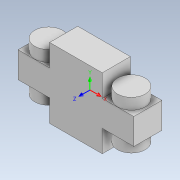
# Autodesk Inventor part: body_inventor
Saved by Autodesk Inventor 2020 (Build 240168000, 168)
## iProperties
Created: 2021-01-07
Part Number: body_inventor
Material: Generic
Document SubType Name: Modeling
Designer: DELL
Density: 1 g/cm^3
Appearance: Default
Author: DELL
Autodesk Inventor part; units mm, degrees
ref_plane "YZ Plane" through (0, 0, 0) normal (1, 0, 0) x (0, 1, 0)
ref_plane "XZ Plane" through (0, 0, 0) normal (0, 1, 0) x (-1, 0, 0)
ref_plane "XY Plane" through (0, 0, 0) normal (0, 0, 1) x (1, 0, 0)
sketch "Sketch4" plane through (0, 0, 0) normal (0, 0, 1) x (1, 0, 0)
  line L0 (75, -100) -> (-75, -100)
  line L1 (-75, -100) -> (-75, 100)
  line L2 (-75, 100) -> (75, 100)
  line L3 (75, 100) -> (75, -100)
  line L4 (75, -100) -> (-75, 100) construction
  line L5 (-75, -100) -> (75, 100) construction
  line L6 (165, -37) -> (-165, -37)
  line L7 (-165, -37) -> (-165, 37)
  line L8 (-165, 37) -> (165, 37)
  line L9 (165, 37) -> (165, -37)
  line L10 (165, -37) -> (-165, 37) construction
  line L11 (-165, -37) -> (165, 37) construction
  point P0 (0, 0)
  point P1 (0, 0)
  point P2 (0, 0)
  point P3 (75, 37)
  point P4 (-75, 37)
  point P5 (-75, -37)
  point P6 (75, -37)
  dimension "d17" = 74
  dimension "d18" = 330
  dimension "d19" = 150
  dimension "d20" = 200
  constraints: 24 end point, 5 midpoint, 4 parallel, 2 horizontal, 2 perpendicular, 1 coincident
  measures "d17" distance of L8.end L6.start
  measures "d18" distance of L6.start L6.end
  measures "d19" distance of L0.start L0.end
  measures "d20" distance of L2.end L0.start
extrude "Extrusion4" add sketch "Sketch4" along normal mid plane 80
sketch "Sketch5" plane through (0, 0, 0) normal (0, 1, 0) x (-1, 0, 0)
  circle A0 centre (-118, 0) radius 39.5
  circle A1 centre (118, 0) radius 39.5
  line L0 (75, 40) -> (-75, 40) construction
  line L1 (0, 40) -> (0, -40) construction
  line L2 (-75, -40) -> (75, -40) construction
  line L3 (-165, -40) -> (-165, 40) construction
  line L4 (-165, 0) -> (165, 0) construction
  line L5 (165, -40) -> (165, 40) construction
  point P0 (0, 0)
  dimension "d23" = 79
  dimension "d24" = 236
  constraints: 4 end point, 4 midpoint, 2 centre point, 1 equal radius, 1 point on line, 1 symmetric about line
  measures "d23" diameter of A0
  measures "d24" distance of A1.centre A0.centre
extrude "Extrusion5" add sketch "Sketch5" along normal mid plane 137.5
sketch "Sketch6" plane through (0, 0, 0) normal (0, 0, 1) x (1, 0, 0)
  line L0 (142, 27) -> (-142, 27)
  line L1 (-142, 27) -> (-142, -27)
  line L2 (-142, -27) -> (142, -27)
  line L3 (142, -27) -> (142, 27)
  line L4 (142, 27) -> (-142, -27) construction
  line L5 (-142, 27) -> (142, -27) construction
  line L6 (-65, 90) -> (65, 90)
  line L7 (65, 90) -> (65, -90)
  line L8 (65, -90) -> (-65, -90)
  line L9 (-65, -90) -> (-65, 90)
  line L10 (-65, 90) -> (65, -90) construction
  line L11 (65, 90) -> (-65, -90) construction
  line L12 (75, -100) -> (-75, -100) projected
  line L13 (-75, 37) -> (-75, 100) projected
  line L14 (-165, -37) -> (-165, 37) projected
  line L15 (-75, -37) -> (-165, -37) projected
  point P0 (0, 0)
  point P1 (-65, -27)
  point P2 (65, -27)
  point P3 (65, 27)
  point P4 (-65, 27)
  dimension "d27" = 10
  dimension "d28" = 10
  dimension "d29" = 23
  dimension "d30" = 10
  constraints: 24 end point, 4 midpoint, 4 parallel, 2 horizontal, 2 perpendicular
  measures "d27" distance between parallel lines of L12 L8
  measures "d28" distance between parallel lines of L13 L9
  measures "d29" distance between parallel lines of L14 L1
  measures "d30" distance between parallel lines of L15 L2
extrude "Extrusion6" cut sketch "Sketch6" along normal mid plane 60
body "Solid1"
body "Solid2"
